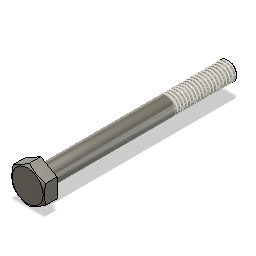
WiFiCam Case (with camera) (Autodesk Fusion 360 archive; units mm, degrees)
design "Hex Head Bolt JIS B 1180 - M4 x 0.7 x 40 - A Steel 4.6 Plain"
description: Hex Head Bolt JIS B 1180 - M4 x 0.7 x 40 - A
Autodesk Fusion 360 part; units mm, degrees
sketch "Sketch1" plane through (0, 0, 0) normal (0, 1, 0) x (1, 0, 0)
  line L0 (-2, 0) -> (-2, 40)
  line L1 (-2, 40) -> (0, 40)
  line L2 (0, 40) -> (0, -3.2)
  line L3 (-2.94, -0.4) -> (-4.0425, -0.4)
  line L4 (-4.0425, -0.4) -> (-4.0425, -2.7858)
  line L5 (-2.94, -0.4) -> (-2.54, 0)
  line L6 (-2.54, 0) -> (-2, 0)
  line L7 (0, -3.2) -> (-3.325, -3.2)
  line L8 (-4.0425, -2.7858) -> (-3.325, -3.2)
  dimension "d81" = 8.085
  dimension "d122" = 135
  dimension "d123" = 0.4
  dimension "d125" = 5.88
  dimension "d127" = 40
  dimension "d149" = 4
  dimension "d156" = 2.8
  dimension "d157" = 30
  dimension "d158" = 6.65
  constraint perpendicular L0 L1
  constraint perpendicular L0 L3
  constraint vertical L0
  constraint vertical L2
  constraint parallel L2 L4
  constraint coincident L2 L7.start
  constraint perpendicular L0 L6
  constraint coincident origin L6
  constraint coincident L0.end L1.start
  constraint perpendicular L2 L7
  constraint coincident origin L2
  measures "d122" angle of L3 L5
  measures "d123" distance of L3 L6
  measures "d127" distance of L1 L6
  measures "d156" distance of L3.end L7
  measures "d157" angle of L7 L8
revolve "Revolve1" add sketch "Sketch1" angle 360 about axis through (0, 0, -40) along (0, 0, 1)
sketch "Sketch8" plane through (0, 0, 3.2) normal (0, 0, 1) x (1, 0, 0)
  line L0 (0, 0) -> (-3.5, 0) construction
  line L1 (-3.5, -2.0228) -> (-3.5, 2.0228)
  circle A0 centre (0, 0) radius 3.325
  circle A1 centre (0, 0) radius 4.0425
  dimension "d114" = 3.5
  constraint coincident L0.start A0.centre
  constraint horizontal L0
  constraint perpendicular L0 L1
  constraint coincident L1.end A1
  constraint coincident L0.end L1
  constraint coincident L1.start A1
  measures "d114" distance of L0.start L1
extrude "Extrude5" cut sketch "Sketch8" against normal blind 2.8 contours L1 A1 picked at (-3.5875, 0.4927)
pattern_circular "C-Pattern2" count 6 over 360 about axis through (0, 0, 1.75) along (0, 0, 1) of "Extrude5"
thread "Thread2" "ISO Metric profile 4.0 M4x0.7 6g" major diameter 3.908 minor diameter 3.111 pitch 0.7 angle 60 resizes the face on face at (-1.9901, 0.1991, -26.6667) from (0, 0, -26.4) to (0, 0, -40)
fillet "Fillet6" radius 0.2 1 edges at (1.954, 0, 0)
sketch "Sketch15" plane through (0, 0, 0) normal (0, 1, 0) x (1, 0, 0)
  line L0 (-2.04, 40) -> (-2.04, 39.5706)
  line L1 (-2.04, 39.5706) -> (-1.5706, 40)
  line L2 (0, 40) -> (0, -3.2)
  line L3 (-2.04, 40) -> (0, 40)
  dimension "d152" = 2.04
  dimension "d153" = 1.5706
  dimension "d154" = 0.4294
  constraint coincident L2.start L3.end
  constraint perpendicular L2 L3
  constraint coincident L1.end L3
  constraint perpendicular L0 L3
  measures "d152" horizontal distance of origin L0.start
  measures "d153" horizontal distance of origin L1.end
  measures "d154" distance of L0.start L0.end
revolve "Revolve4" cut sketch "Sketch15" angle 360 about axis through (0, 0, 1.75) along (0, 0, 1)
equation "adsk_nomlen = 40.00 mm"
equation "adsk_headh = 2.80 mm"
equation "adsk_headdia = 8.085 mm"
equation "adsk_nomdia = 4.00 mm"
equation "d81 = adsk_headdia"
equation "d89 = -adsk_headh"
equation "adsk_waflat = 7.00 mm"
equation "d114 = adsk_waflat / 2"
equation "adsk_thrlen = 14.00 mm"
equation "adsk_chamang2 = 30.00 deg"
equation "adsk_midfillet = 0.20 mm"
equation "d123 = adsk_necklen"
equation "adsk_necklen = 0.40 mm"
equation "d125 = adsk_neckdia"
equation "adsk_neckdia = 5.88 mm"
equation "d127 = adsk_nomlen"
equation "d138 = adsk_midfillet"
equation "d140 = adsk_thrlen - adsk_necklen"
equation "adsk_endpointdia = 3.14117 mm"
equation "adsk_startlen = 0.429415 mm"
equation "d149 = adsk_nomdia"
equation "d152 = adsk_nomdia * 0.51"
equation "d153 = adsk_endpointdia / 2"
equation "d154 = adsk_startlen"
equation "d156 = adsk_headh"
equation "d157 = adsk_chamang2"
equation "d158 = adsk_waflat * 0.95"
